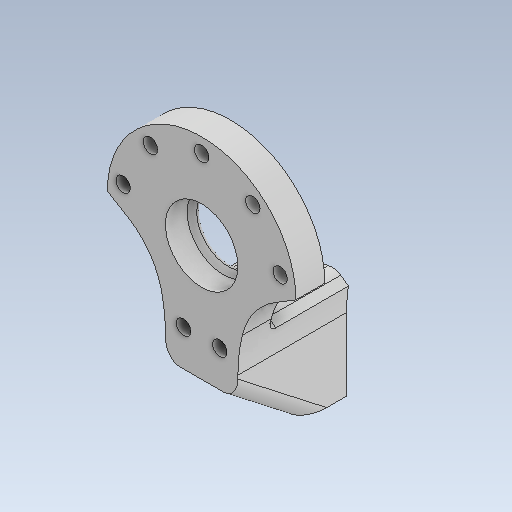
# Autodesk Inventor part: bone_upper_3
Saved by Autodesk Inventor 2020 (Build 240168000, 168)
## iProperties
Created: 2019-05-04
Part Number: bone_upper_3
Material: Generic
Document SubType Name: Modeling
Designer: psrob
Density: 1 g/cm^3
Appearance: Default
Author: psrob
Autodesk Inventor part; units mm, degrees
ref_plane "YZ Plane" through (0, 0, 0) normal (1, 0, 0) x (0, 1, 0)
ref_plane "XZ Plane" through (0, 0, 0) normal (0, 1, 0) x (-1, 0, 0)
ref_plane "XY Plane" through (0, 0, 0) normal (0, 0, 1) x (1, 0, 0)
sketch "Sketch1" plane through (0, 0, 0) normal (0, 0, 1) x (1, 0, 0)
  circle A0 centre (3, 63) radius 3 projected
  circle A1 centre (3, 63) radius 8
  line L0 (6, 0) -> (6, 50) projected
  line L1 (0, 0) -> (6, 0) projected
  line L2 (6, 0) -> (6, 50) projected
  line L3 (0, 50) -> (6, 50) projected
  line L4 (0, 0) -> (0, 50) projected
  line L5 (6, 50) -> (8, 50)
  line L6 (8, 50) -> (-2, 50)
  line L7 (-2, 50) -> (-2, 40)
  line L8 (-2, 40) -> (8, 40)
  line L9 (8, 40) -> (8, 50)
  line L10 (3, 63) -> (10.191, 59.4944)
  line L11 (3, 63) -> (-4.191, 59.4944)
  arc A2 (-2, 50) -> (-4.191, 59.4944) centre (-23.6667, 50) ccw
  arc A3 (10.191, 59.4944) -> (8, 50) centre (29.6667, 50) ccw
  dimension "d0" = 16
  dimension "d1" = 2
  dimension "d2" = 10
  dimension "d3" = 10
  constraints: 14 end point, 6 point on circle, 4 line through centre, 3 centre point, 2 parallel, 2 perpendicular, 1 coincident, 1 horizontal
  measures "d0" diameter of A1
  measures "d1" distance of L0.end L5.end
  measures "d2" distance of L8.end L7.end
  measures "d3" distance of L7.end L6.end
extrude "Extrusion1" add sketch "Sketch1" along normal blind 14 contours A0 L10 L11 | A0 L11 A1 L10 | L11 L10 A0 | A0 L10 A1 L11 | A1 A3 L5 L3 L6 A2 | L6 L4 L8 L7 | L9 L8 L0 L5 | L3 L0 L8 L4
sketch "Sketch2" plane through (0, 0, 0) normal (0, 0, -1) x (-1, 0, 0)
  circle A0 centre (-3, 63) radius 3 projected
  circle A1 centre (-3, 63) radius 9
  point P0 (0, 0)
  dimension "d6" = 18
  constraints: 1 centre point, 1 coincident
  measures "d6" diameter of A1
extrude "Extrusion2" cut sketch "Sketch2" against normal blind 8 contours A0 | A1
thicken "Thicken1" operation add thickness 2 both sides no extend neighbours yes toward (0, 0, -1) faces at (4.7053, 63.6847, 14)
chamfer "Chamfer1" distance 3 angle 45 2 edges at (-2.9096, 56.212, 4) (8.9096, 56.212, 4)
fillet "Fillet1" radius 1 3 edges at (-1.3004, 53.9661, 8) (3, 54, 8) (7.3004, 53.9661, 8)
sketch "Sketch3" plane through (0, 0, 0) normal (0, 0, -1) x (-1, 0, 0)
  line L0 (2, 40) -> (2, 49.6056)
  line L1 (0, 40) -> (-6, 40)
  line L2 (2, 40) -> (0, 40)
  line L3 (-6, 40) -> (-8, 40)
  line L4 (-8, 49.6056) -> (-8, 40)
  arc A0 (2.2505, 53.2853) -> (2, 50) centre (23.6667, 50) ccw
  line L5 (-8.2505, 53.2853) -> (-6.3503, 54.6468)
  arc A1 (-8, 50) -> (-8.2505, 53.2853) centre (-29.6667, 50) ccw
  line L6 (-8, 40) -> (-8, 50)
  line L7 (2, 40) -> (-8, 40)
  line L8 (2, 50) -> (2, 40)
  arc A2 (2.2505, 53.2853) -> (2, 50) centre (23.6667, 50) ccw
  line L9 (0.3503, 54.6468) -> (2.2505, 53.2853)
  arc A3 (-6.3503, 54.6468) -> (0.3503, 54.6468) centre (-3, 63) ccw
  line L10 (-6, 0) -> (0, 0)
  line L11 (0, 0) -> (0, 50)
  line L12 (-6, 50) -> (0, 50)
  line L13 (-6, 0) -> (-6, 50)
  point P0 (2.2505, 53.2853)
  point P1 (2, 50)
extrude "Extrusion3" add sketch "Sketch3" along normal blind 3 contours L2 L11 L12 L13 L3 L4 L6 A1 L5 A3 L9 A0 L8 L0
fillet "Fillet2" radius 2 6 edges at (-0.3897, 54.9863, 7.7131) (-0.3503, 54.6468, -1.5) (-0.3503, 54.6468, 3.5) (6.3897, 54.9863, 7.7131) (6.3503, 54.6468, -1.5) (6.3503, 54.6468, 3.5)
sketch "Sketch4" plane through (0, 0, -3) normal (0, 0, -1) x (-1, 0, 0)
  circle A0 centre (-5.5, 52) radius 1 projected
  circle A1 centre (-0.5, 52) radius 1 projected
  point P0 (0, 0)
extrude "Extrusion4" cut sketch "Sketch4" against normal blind 20
sketch "Sketch6" plane through (-2, 40, 12) normal (-1, 0, 0) x (0, 0, 1)
  line L0 (0, 0) -> (-15, 0) projected
  line L1 (0, 10) -> (0, 0) projected
  line L2 (-15, 10) -> (0, 10) projected
  line L3 (-15, 0) -> (-15, 10) projected
  line L4 (0, 0) -> (0, 7)
  line L5 (0, 10) -> (0, 0) projected
  line L6 (0, 0) -> (-9, 0)
  line L7 (0, 0) -> (-15, 0) projected
  line L8 (-9, 0) -> (0, 7)
  point P0 (-12, -40)
  point P1 (0, 7)
  point P2 (-9, 0)
  dimension "d25" = 7
  dimension "d26" = 9
  constraints: 6 end point, 2 point on line
  measures "d25" distance of L0.start L4.end
  measures "d26" distance of L0.start L6.end
extrude "Extrusion6" cut sketch "Sketch6" against normal blind 20 contours L0 L8 L1
fillet "Fillet3" radius 2 2 edges at (8, 43.5, 7.5) (-2, 43.5, 7.5)
sketch "Sketch7" plane through (0, 40, 3) normal (0, -0.7893522, 0.6139406) x (1, 0, 0)
  line L0 (0, 0) -> (0, 11.4018) projected
  line L1 (6, 0) -> (0, 0) projected
  line L2 (6, 11.4018) -> (6, 0) projected
  line L3 (0, 11.4018) -> (6, 11.4018) projected
  line L4 (6, 0) -> (0, 0) projected
  line L5 (0, 0) -> (6, 11.4018)
  line L6 (0, 11.4018) -> (6, 0)
  circle A0 centre (3, 5.7009) radius 1
  point P0 (0, -26.9257)
  dimension "d30" = 2
  constraints: 4 end point, 1 centre point, 1 midpoint
  measures "d30" diameter of A0
extrude "Extrusion7" cut sketch "Sketch7" against normal blind 6 contours A0 L6 L5 | L5 L6 A0 | A0 L5 L6 | L6 L5 A0
sketch "Sketch8" plane through (3, 63, 12) normal (0, 0, 1) x (1, 0, 0)
  ellipse E0 centre (-3, -13.4663) end of major axis (-3, -16) minor radius 2 (-5, -13.4663) -> (-3, -16) ccw projected
  line L0 (-3, -16) -> (3, -16) projected
  ellipse E1 centre (3, -13.4663) end of major axis (3, -16) minor radius 2 (3, -16) -> (5, -13.4663) ccw projected
  line L1 (5, -13.4663) -> (5, -13) projected
  arc A0 (7.191, -3.5056) -> (5, -13) centre (26.6667, -13) ccw projected
  arc A1 (7.191, -3.5056) -> (-7.191, -3.5056) centre (0, 0) ccw projected
  arc A2 (-5, -13) -> (-7.191, -3.5056) centre (-26.6667, -13) ccw projected
  line L2 (-5, -13) -> (-5, -13.4663) projected
  circle A3 centre (2.5, -11) radius 1 projected
  circle A4 centre (-2.5, -11) radius 1 projected
  circle A5 centre (0, 0) radius 5
  point P0 (-3, -63)
  dimension "d33" = 10
  constraints: 1 centre point, 1 coincident, 2 other
  measures "d33" diameter of A5
extrude "Extrusion8" cut sketch "Sketch8" against normal blind 6 contours A5
sketch "Sketch9" plane through (0, 0, 8) normal (0, 0, -1) x (-1, 0, 0)
  circle A0 centre (-3, 63) radius 5 projected
  circle A1 centre (-3, 63) radius 4
  point P0 (0, 0)
  dimension "d36" = 8
  constraints: 1 centre point, 1 coincident
  measures "d36" diameter of A1
extrude "Extrusion9" add sketch "Sketch9" against normal blind 1
chamfer "Chamfer2" distance 1 angle 45 1 edges at (7, 63, 9)
fillet "Fillet4" radius 0.2 2 edges at (7, 63, 8.0001) (7, 63, 8)
sketch "Sketch11" plane through (3, 63, 12) normal (0, 0, 1) x (1, 0, 0)
  circle A0 centre (0, 0) radius 5 projected
  ellipse E0 centre (-3, -13.3944) end of major axis (-3, -17) minor radius 2 (-5, -13.3944) -> (-3, -17) ccw projected
  line L0 (-5, -13.3944) -> (-5, -13) projected
  arc A1 (-5, -13) -> (-5.5977, -7.9461) centre (-26.6667, -13) ccw projected
  arc A2 (-5.5977, -7.9461) -> (-10.155, -1.7169) centre (-15.3218, -10.2787) ccw projected
  line L1 (-10.155, -1.7169) -> (-13, 0) projected
  arc A3 (13, 0) -> (-13, 0) centre (0, 0) ccw projected
  line L2 (13, 0) -> (10.155, -1.7169) projected
  arc A4 (10.155, -1.7169) -> (5.5977, -7.9461) centre (15.3218, -10.2787) ccw projected
  arc A5 (5.5977, -7.9461) -> (5, -13) centre (26.6667, -13) ccw projected
  line L3 (5, -13) -> (5, -13.3944) projected
  ellipse E1 centre (3, -13.3944) end of major axis (3, -17) minor radius 2 (3, -17) -> (5, -13.3944) ccw projected
  line L4 (3, -17) -> (-3, -17) projected
  circle A6 centre (2.5, -11) radius 1 projected
  circle A7 centre (-2.5, -11) radius 1 projected
  arc A8 (7.191, -3.5056) -> (-7.191, -3.5056) centre (0, 0) ccw projected
  arc A9 (-5, -13) -> (-7.191, -3.5056) centre (-26.6667, -13) ccw projected
  arc A10 (7.191, -3.5056) -> (5, -13) centre (26.6667, -13) ccw projected
  circle A11 centre (0, 11) radius 1 projected
  circle A12 centre (-7.0707, 8.4265) radius 1 projected
  circle A13 centre (7.0707, 8.4265) radius 1 projected
  circle A14 centre (-10.8329, 1.9101) radius 1 projected
  circle A15 centre (10.8329, 1.9101) radius 1 projected
  point P0 (-3, -63)
  constraints: 2 other
extrude "Extrusion11" add sketch "Sketch11" against normal blind 4 contours A2 L1 A3 L2 A4 A10 A8 A9 | A11 | A12 | A13 | A14 | A15
sketch "Sketch12" plane through (0, 47, 12) normal (0, 0, 1) x (1, 0, 0)
  circle A0 centre (3, 27) radius 1 projected
  circle A1 centre (10.0707, 24.4265) radius 1 projected
  circle A2 centre (13.8329, 17.9101) radius 1 projected
  circle A3 centre (-4.0707, 24.4265) radius 1 projected
  circle A4 centre (-7.8329, 17.9101) radius 1 projected
  point P0 (0, -47)
extrude "Extrusion12" cut sketch "Sketch12" against normal blind 4
body "Solid1"
